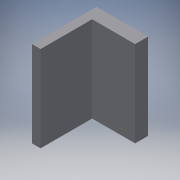
# Autodesk Inventor part: commutator_attatchment_pulley_bridge
Saved by Autodesk Inventor 2016 (Build 200138000, 138)
## iProperties
Created: 2016-09-29
Part Number: commutator_attatchment_pulley_bridge
Material: Generic
Document SubType Name: Modeling
Designer: ajar021
Density: 1 g/cm^3
Appearance: Default
Author: ajar021
Autodesk Inventor part; units mm, degrees
ref_plane "YZ Plane" through (0, 0, 0) normal (1, 0, 0) x (0, 1, 0)
ref_plane "XZ Plane" through (0, 0, 0) normal (0, 1, 0) x (-1, 0, 0)
ref_plane "XY Plane" through (0, 0, 0) normal (0, 0, 1) x (1, 0, 0)
sketch "Sketch1" plane through (0, 0, 0) normal (0, 0, 1) x (1, 0, 0)
  line L0 (6, -10) -> (6, 10) projected
  line L1 (6, 10) -> (-6, 10) projected
  line L2 (-6, 10) -> (-6, -10) projected
  line L3 (-6, -10) -> (6, -10) projected
  point P0 (0, 0)
extrude "Extrusion1" add sketch "Sketch1" along normal blind 3
sketch "Sketch2" plane through (0, 0, 3) normal (0, 0, 1) x (1, 0, 0)
  line L0 (6, 10) -> (-6, 10) projected
  line L1 (-6, 10) -> (-6, -10) projected
  line L2 (-6, -10) -> (6, -10) projected
  line L3 (-6, 10) -> (-4, 10)
  line L4 (-4, 10) -> (-4, -10)
  line L5 (-6, -10) -> (-6, 10)
  point P0 (0, 0)
  dimension "d2" = 2
  constraints: 6 end point, 2 point on line, 1 collinear, 1 perpendicular
  measures "d2" distance of L0.end L3.end
extrude "Extrusion2" add sketch "Sketch2" along normal blind 12
body "Solid1"
